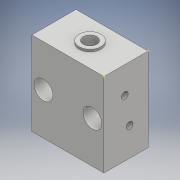
# Autodesk Inventor part: コガネイ_BDA16x5
Saved by Autodesk Inventor 2018 (Build 220112000, 112)
## iProperties
Created: 2018-04-18
Part Number: コガネイ_BDA16x5
Material: 一般
Document SubType Name: Modeling
Designer: Take
Density: 1 g/cm^3
Appearance: 既定
Author: Take
Autodesk Inventor part; units mm, degrees
ref_plane "YZ Plane" through (0, 0, 0) normal (1, 0, 0) x (0, 1, 0)
ref_plane "XZ Plane" through (0, 0, 0) normal (0, 1, 0) x (-1, 0, 0)
ref_plane "XY Plane" through (0, 0, 0) normal (0, 0, 1) x (1, 0, 0)
sketch "スケッチ1" plane through (0, 0, 0) normal (0, 1, 0) x (-1, 0, 0)
  line L0 (0, 0) -> (33, 0)
  line L1 (33, 0) -> (33, -38.3)
  line L2 (33, -38.3) -> (0, -38.3)
  line L3 (0, -38.3) -> (0, 0)
  dimension "d0" = 33
  dimension "d1" = 38.3
  constraints: 8 end point, 2 parallel, 1 horizontal, 1 perpendicular
  measures "d0" distance of L1.end L2.end
  measures "d1" distance of L0.end L1.end
extrude "押し出し1" add sketch "スケッチ1" along normal blind 20.2
sketch "スケッチ2" plane through (0, 20.2, 0) normal (0, 1, 0) x (1, 0, 0)
  line L0 (-33, 38.3) -> (-33, 0) projected
  line L1 (-33, 19.15) -> (0, 19.15)
  line L2 (0, 0) -> (0, 38.3) projected
  point P0 (-27.7, 19.15)
  point P1 (-5.3, 19.15)
  dimension "d4" = 5.3
  dimension "d5" = 5.3
  constraints: 2 end point, 2 midpoint, 2 point on line
  measures "d4" distance from line of L0 point (-27.7, 19.15)
  measures "d5" distance from line of L2 point (-5.3, 19.15)
sketch "スケッチ3" plane through (0, 20.2, 0) normal (0, 1, 0) x (1, 0, 0)
  point P0 (0, 0)
sketch "スケッチ4" plane through (0, 20.2, 0) normal (0, 1, 0) x (1, 0, 0)
  circle A0 centre (-5.3, 19.15) radius 4.3
  circle A1 centre (-27.7, 19.15) radius 4.3
  point P0 (0, 0)
  dimension "d6" = 8.6
  dimension "d7" = 8.6
  constraints: 2 centre point
  measures "d6" diameter of A0
  measures "d7" diameter of A1
hole "穴1" at (-5.3, 20.2, -19.15) direction (0, -1, 0) diameter 8.6 end through all
hole "穴2" at (-27.7, 20.2, -19.15) direction (0, -1, 0) diameter 8.6 end through all
sketch "スケッチ5" plane through (-33, 0, 0) normal (0, 0, 1) x (1, 0, 0)
  line L0 (33, 20.2) -> (0, 20.2) projected
  line L1 (16.5, 20.2) -> (16.5, 0)
  circle A0 centre (16.5, 10.1) radius 5
  circle A1 centre (16.5, 10.1) radius 3.1
  point P0 (33, 0)
  dimension "d22" = 10
  dimension "d23" = 6.2
  constraints: 2 centre point, 2 coincident, 2 end point, 2 midpoint, 1 vertical
  measures "d22" diameter of A0
  measures "d23" diameter of A1
sketch "スケッチ6" plane through (0, 0, 0) normal (1, 0, 0) x (0, 0, -1)
  line L0 (0, 0) -> (38.3, 0) projected
  line L1 (12.25, 0) -> (12.25, 20.2)
  line L2 (0, 20.2) -> (38.3, 20.2) projected
  line L3 (25.25, 0) -> (25.25, 20.2)
  point P0 (12.25, 9.5)
  point P1 (25.25, 11.7)
  dimension "d26" = 9.5
  dimension "d27" = 8.5
  constraints: 6 point on line, 4 end point, 1 perpendicular, 1 vertical
  measures "d26" distance from line of L0 point (12.25, 9.5)
  measures "d27" distance from line of L2 point (25.25, 11.7)
sketch "スケッチ7" plane through (0, 0, 0) normal (1, 0, 0) x (0, 0, -1)
  point P0 (0, 0)
hole "穴3" at (0, 9.5, -12.25) at (0, 11.7, -25.25) direction (-1, 0, 0) diameter 3.1 depth 6 tip angle 118
extrude "押し出し3" add sketch "スケッチ5" along normal blind 1 contours A0 L1 A1 | L1 A1 A0
sketch "スケッチ8" plane through (-33, 0, 0) normal (0, 0, 1) x (1, 0, 0)
  line L0 (0, 20.2) -> (33, 20.2) projected
  line L1 (16.5, 20.2) -> (16.5, 0)
  line L2 (33, 0) -> (0, 0) projected
  point P0 (16.5, 10.1)
  constraints: 3 midpoint, 2 end point
hole "穴4" at (-16.5, 10.1, 0) direction (0, 0, -1) diameter 6.2 depth 10
